Autodesk Inventor part; units mm, degrees
(part 2 of 2)
sketch "スケッチ10" plane through (0, 0, 0) normal (0, 0, 1) x (1, 0, 0)
  arc A0 (-142.506418, -9.086216) -> (-131.660668, -10.24148) centre (-136.463592, -3.843674) ccw
  line L0 (-142.506418, -9.086216) -> (-153.239213, 3.284961)
  arc A1 (-152.436991, 13.246431) -> (-153.239213, 3.284961) centre (-147.951739, 7.872185) ccw
  line L1 (-152.436991, 13.246431) -> (-136.850058, 26.255011)
  arc A2 (-136.058454, 26.82081) -> (-136.850058, 26.255011) centre (-132.685182, 21.264639) ccw
  line L2 (-136.058454, 26.82081) -> (-64.095126, 70.511318)
  arc A3 (-60.233181, 71.528052) -> (-64.095126, 70.511318) centre (-60.449397, 64.50638) ccw
  line L3 (-60.233181, 71.528052) -> (-56.416161, 71.410515)
  line L4 (-56.416161, 71.410515) -> (-62.310529, 66.98553)
  arc A4 (-62.310529, 66.98553) -> (-58.588264, 62.02723) centre (-60.449397, 64.50638) ccw
  line L5 (-58.588264, 62.02723) -> (-46.496021, 71.105048)
  line L6 (-46.496021, 71.105048) -> (-44.232954, 71.035362)
  arc A5 (-41.268818, 70.277554) -> (-44.232954, 71.035362) centre (-44.44917, 64.013691) ccw
  line L7 (-41.268818, 70.277554) -> (-66.303447, 51.483704)
  arc A6 (-66.303447, 51.483704) -> (-62.581181, 46.525404) centre (-64.442314, 49.004554) ccw
  line L8 (-62.581181, 46.525404) -> (-37.546552, 65.319255)
  arc A7 (-40.231602, 58.395617) -> (-37.546552, 65.319255) centre (-44.44917, 64.013691) ccw
  line L9 (-40.231602, 58.395617) -> (-131.660668, -10.24148)
  circle A8 centre (-147.951739, 7.872185) radius 3
  circle A9 centre (-136.463592, -3.843674) radius 3
  circle A10 centre (-84.115857, 33.578871) radius 3
  circle A11 centre (-112.106259, 12.566079) radius 3
  circle A12 centre (-77.811872, 54.579424) radius 3
  circle A13 centre (-132.685182, 21.264639) radius 3
  circle A14 centre (-105.248527, 37.922031) radius 3
  arc A15 (-133.54471, 2.112846) -> (-133.114093, 1.134364) centre (-132.555844, 1.964037) ccw
  arc A16 (-130.83606, -1.762597) -> (-133.114093, 1.134364) centre (-136.463592, -3.843674) ccw
  arc A17 (-130.83606, -1.762597) -> (-129.297772, -2.215477) centre (-129.898137, -1.415751) ccw
  line L10 (-129.297772, -2.215477) -> (-116.789492, 7.174667)
  arc A18 (-116.789492, 7.174667) -> (-116.635058, 8.630348) centre (-117.389857, 7.974392) ccw
  arc A19 (-117.147544, 9.312551) -> (-116.635058, 8.630348) centre (-112.106259, 12.566079) ccw
  arc A20 (-117.147544, 9.312551) -> (-118.117598, 9.761832) centre (-117.987758, 8.770297) ccw
  line L11 (-118.117598, 9.761832) -> (-131.933702, 7.95264)
  arc A21 (-131.933702, 7.95264) -> (-132.792729, 7.109914) centre (-131.803863, 6.961105) ccw
  line L12 (-132.792729, 7.109914) -> (-133.54471, 2.112846)
  arc A22 (-88.79909, 28.187458) -> (-88.644656, 29.643139) centre (-89.399456, 28.987184) ccw
  arc A23 (-89.943579, 32.151404) -> (-88.644656, 29.643139) centre (-84.115857, 33.578871) ccw
  arc A24 (-89.943579, 32.151404) -> (-90.713554, 32.89302) centre (-90.914866, 31.913493) ccw
  line L13 (-90.713554, 32.89302) -> (-99.456074, 34.689773)
  arc A25 (-99.456074, 34.689773) -> (-100.45612, 34.311929) centre (-99.657386, 33.710245) ccw
  arc A26 (-104.181599, 32.017655) -> (-100.45612, 34.311929) centre (-105.248527, 37.922031) ccw
  arc A27 (-104.181599, 32.017655) -> (-104.969096, 31.29467) centre (-104.003778, 31.033592) ccw
  line L14 (-104.969096, 31.29467) -> (-108.524419, 18.149127)
  arc A28 (-108.524419, 18.149127) -> (-108.208695, 17.127767) centre (-107.559102, 17.888049) ccw
  arc A29 (-107.062861, 15.816331) -> (-108.208695, 17.127767) centre (-112.106259, 12.566079) ccw
  arc A30 (-107.062861, 15.816331) -> (-105.621929, 15.558314) centre (-106.222295, 16.35804) ccw
  line L15 (-105.621929, 15.558314) -> (-88.79909, 28.187458)
  line L16 (-130.745103, 12.142434) -> (-123.324226, 13.114183)
  arc A31 (-123.324226, 13.114183) -> (-123.064726, 15.026812) centre (-123.454066, 14.105718) ccw
  line L17 (-123.064726, 15.026812) -> (-127.63835, 16.96005)
  arc A32 (-127.63835, 16.96005) -> (-128.693046, 16.785482) centre (-128.02769, 16.038956) ccw
  arc A33 (-130.949084, 15.521298) -> (-128.693046, 16.785482) centre (-132.685182, 21.264639) ccw
  arc A34 (-130.949084, 15.521298) -> (-131.6486, 14.712884) centre (-130.659734, 14.564075) ccw
  line L18 (-131.6486, 14.712884) -> (-131.863809, 13.282778)
  arc A35 (-131.863809, 13.282778) -> (-130.745103, 12.142434) centre (-130.874943, 13.133969) ccw
  arc A36 (-126.690727, 21.522538) -> (-127.791923, 24.736817) centre (-132.685182, 21.264639) ccw
  arc A37 (-126.690727, 21.522538) -> (-126.080991, 20.644427) centre (-125.691651, 21.565521) ccw
  line L19 (-126.080991, 20.644427) -> (-117.15309, 16.870668)
  arc A38 (-117.15309, 16.870668) -> (-116.098395, 17.045236) centre (-116.763751, 17.791763) ccw
  arc A39 (-113.173186, 18.470456) -> (-116.098395, 17.045236) centre (-112.106259, 12.566079) ccw
  arc A40 (-113.173186, 18.470456) -> (-112.38569, 19.19344) centre (-113.351007, 19.454519) ccw
  line L20 (-112.38569, 19.19344) -> (-108.830366, 32.338983)
  arc A41 (-108.830366, 32.338983) -> (-109.14609, 33.360343) centre (-109.795684, 32.600062) ccw
  arc A42 (-110.586613, 35.182536) -> (-109.14609, 33.360343) centre (-105.248527, 37.922031) ccw
  arc A43 (-110.586613, 35.182536) -> (-111.995259, 35.580749) centre (-111.476294, 34.725953) ccw
  line L21 (-111.995259, 35.580749) -> (-127.495344, 26.170308)
  arc A44 (-127.495344, 26.170308) -> (-127.791923, 24.736817) centre (-126.976379, 25.315513) ccw
  arc A45 (-71.858452, 55.325612) -> (-70.160292, 54.741689) centre (-70.866216, 55.449977) ccw
  arc A46 (-69.305274, 55.482332) -> (-70.160292, 54.741689) centre (-64.442314, 49.004554) ccw
  line L22 (-69.305274, 55.482332) -> (-66.550527, 57.55036)
  arc A47 (-66.550527, 57.55036) -> (-66.414464, 59.026602) centre (-67.150892, 58.350086) ccw
  arc A48 (-67.802662, 61.109398) -> (-66.414464, 59.026602) centre (-60.449397, 64.50638) ccw
  arc A49 (-67.802662, 61.109398) -> (-69.229438, 61.544813) centre (-68.710473, 60.690017) ccw
  line L23 (-69.229438, 61.544813) -> (-72.622035, 59.485093)
  arc A50 (-72.622035, 59.485093) -> (-72.918613, 58.051601) centre (-72.10307, 58.630298) ccw
  arc A51 (-71.858452, 55.325612) -> (-72.918613, 58.051601) centre (-77.811872, 54.579424) ccw
  arc A52 (-100.058689, 42.827701) -> (-100.355268, 41.394209) centre (-99.539724, 41.972905) ccw
  arc A53 (-99.420805, 39.349498) -> (-100.355268, 41.394209) centre (-105.248527, 37.922031) ccw
  arc A54 (-99.420805, 39.349498) -> (-98.650829, 38.607882) centre (-98.449518, 39.587409) ccw
  line L24 (-98.650829, 38.607882) -> (-89.908309, 36.81113)
  arc A55 (-89.908309, 36.81113) -> (-88.908264, 37.188973) centre (-89.706998, 37.790657) ccw
  arc A56 (-85.020123, 39.510338) -> (-88.908264, 37.188973) centre (-84.115857, 33.578871) ccw
  arc A57 (-85.020123, 39.510338) -> (-84.213055, 40.211408) centre (-85.170834, 40.498916) ccw
  line L25 (-84.213055, 40.211408) -> (-81.545787, 49.096917)
  arc A58 (-81.545787, 49.096917) -> (-81.833323, 50.126568) centre (-82.503565, 49.384425) ccw
  arc A59 (-83.149958, 51.839928) -> (-81.833323, 50.126568) centre (-77.811872, 54.579424) ccw
  arc A60 (-83.149958, 51.839928) -> (-84.558604, 52.238141) centre (-84.039639, 51.383346) ccw
  line L26 (-84.558604, 52.238141) -> (-100.058689, 42.827701)
  arc A61 (-137.554519, 17.758994) -> (-139.006826, 17.942469) centre (-138.366076, 17.174719) ccw
  line L27 (-139.006826, 17.942469) -> (-143.139417, 14.493481)
  arc A62 (-143.139417, 14.493481) -> (-143.180301, 12.994038) centre (-142.498667, 13.725731) ccw
  arc A63 (-141.858325, 11.317516) -> (-143.180301, 12.994038) centre (-147.951739, 7.872185) ccw
  arc A64 (-141.858325, 11.317516) -> (-140.857998, 10.818171) centre (-140.987838, 11.809706) ccw
  line L28 (-140.857998, 10.818171) -> (-136.934628, 11.331928)
  arc A65 (-136.934628, 11.331928) -> (-136.075602, 12.174654) centre (-137.064468, 12.323463) ccw
  line L29 (-136.075602, 12.174654) -> (-135.604064, 15.308119)
  arc A66 (-135.604064, 15.308119) -> (-136.03468, 16.286601) centre (-136.59293, 15.456928) ccw
  arc A67 (-137.554519, 17.758994) -> (-136.03468, 16.286601) centre (-132.685182, 21.264639) ccw
  arc A68 (-138.19969, 1.899667) -> (-137.500173, 2.708082) centre (-138.489039, 2.856891) ccw
  line L30 (-137.500173, 2.708082) -> (-137.004522, 6.001791)
  arc A69 (-137.004522, 6.001791) -> (-138.123227, 7.142135) centre (-137.993388, 6.1506) ccw
  line L31 (-138.123227, 7.142135) -> (-140.33864, 6.852031)
  arc A70 (-140.33864, 6.852031) -> (-141.176668, 6.111957) centre (-140.2088, 5.860496) ccw
  arc A71 (-144.061428, 2.05278) -> (-141.176668, 6.111957) centre (-147.951739, 7.872185) ccw
  arc A72 (-144.061428, 2.05278) -> (-144.261023, 0.566118) centre (-143.505669, 1.221436) ccw
  line L32 (-144.261023, 0.566118) -> (-143.125657, -0.742563)
  arc A73 (-143.125657, -0.742563) -> (-141.526488, -0.623878) centre (-142.370304, -0.087245) ccw
  arc A74 (-138.19969, 1.899667) -> (-141.526488, -0.623878) centre (-136.463592, -3.843674) ccw
  arc A75 (-76.907606, 48.647957) -> (-74.152214, 49.824752) centre (-77.811872, 54.579424) ccw
  arc A76 (-76.907606, 48.647957) -> (-77.714673, 47.946886) centre (-76.756895, 47.659379) ccw
  line L33 (-77.714673, 47.946886) -> (-80.381942, 39.061377)
  arc A77 (-80.381942, 39.061377) -> (-80.094406, 38.031727) centre (-79.424164, 38.77387) ccw
  arc A78 (-79.072459, 36.829123) -> (-80.094406, 38.031727) centre (-84.115857, 33.578871) ccw
  arc A79 (-79.072459, 36.829123) -> (-77.631528, 36.571106) centre (-78.231893, 37.370832) ccw
  line L34 (-77.631528, 36.571106) -> (-70.457765, 41.956551)
  arc A80 (-70.457765, 41.956551) -> (-70.331118, 43.4429) centre (-71.058131, 42.756277) ccw
  arc A81 (-72.542276, 49.029257) -> (-70.331118, 43.4429) centre (-64.442314, 49.004554) ccw
  arc A82 (-72.542276, 49.029257) -> (-74.152214, 49.824752) centre (-73.542271, 49.032306) ccw
  arc A83 (-117.147544, 9.312551) -> (-116.635058, 8.630348) centre (-112.106259, 12.566079) ccw
  arc A84 (-116.789492, 7.174667) -> (-116.635058, 8.630348) centre (-117.389857, 7.974392) ccw
  line L35 (-116.789492, 7.174667) -> (-129.297772, -2.215477)
  arc A85 (-130.83606, -1.762597) -> (-129.297772, -2.215477) centre (-129.898137, -1.415751) ccw
  arc A86 (-130.83606, -1.762597) -> (-133.114093, 1.134364) centre (-136.463592, -3.843674) ccw
  arc A87 (-133.54471, 2.112846) -> (-133.114093, 1.134364) centre (-132.555844, 1.964037) ccw
  line L36 (-133.54471, 2.112846) -> (-132.792729, 7.109914)
  arc A88 (-131.933702, 7.95264) -> (-132.792729, 7.109914) centre (-131.803863, 6.961105) ccw
  line L37 (-131.933702, 7.95264) -> (-118.117598, 9.761832)
  arc A89 (-117.147544, 9.312551) -> (-118.117598, 9.761832) centre (-117.987758, 8.770297) ccw
  arc A90 (-142.910454, 11.125713) -> (-145.546046, 13.368787) centre (-147.951739, 7.872185) ccw
  arc A91 (-145.664062, 15.139683) -> (-145.546046, 13.368787) centre (-145.145097, 14.284888) ccw
  line L38 (-145.664062, 15.139683) -> (-139.431914, 18.923356)
  arc A92 (-138.023268, 18.525143) -> (-139.431914, 18.923356) centre (-138.912949, 18.068561) ccw
  arc A93 (-138.023268, 18.525143) -> (-136.03468, 16.286601) centre (-132.685182, 21.264639) ccw
  arc A94 (-135.604064, 15.308119) -> (-136.03468, 16.286601) centre (-136.59293, 15.456928) ccw
  line L39 (-135.604064, 15.308119) -> (-136.075602, 12.174654)
  arc A95 (-136.934628, 11.331928) -> (-136.075602, 12.174654) centre (-137.064468, 12.323463) ccw
  line L40 (-136.934628, 11.331928) -> (-141.9404, 10.676432)
  arc A96 (-142.910454, 11.125713) -> (-141.9404, 10.676432) centre (-142.07024, 11.667967) ccw
  arc A97 (-110.586613, 35.182536) -> (-109.14609, 33.360343) centre (-105.248527, 37.922031) ccw
  arc A98 (-108.830366, 32.338983) -> (-109.14609, 33.360343) centre (-109.795684, 32.600062) ccw
  line L41 (-108.830366, 32.338983) -> (-112.38569, 19.19344)
  arc A99 (-113.173186, 18.470456) -> (-112.38569, 19.19344) centre (-113.351007, 19.454519) ccw
  arc A100 (-113.173186, 18.470456) -> (-116.098395, 17.045236) centre (-112.106259, 12.566079) ccw
  arc A101 (-117.15309, 16.870668) -> (-116.098395, 17.045236) centre (-116.763751, 17.791763) ccw
  line L42 (-117.15309, 16.870668) -> (-126.080991, 20.644427)
  arc A102 (-126.690727, 21.522538) -> (-126.080991, 20.644427) centre (-125.691651, 21.565521) ccw
  arc A103 (-126.690727, 21.522538) -> (-127.791923, 24.736817) centre (-132.685182, 21.264639) ccw
  arc A104 (-127.495344, 26.170308) -> (-127.791923, 24.736817) centre (-126.976379, 25.315513) ccw
  line L43 (-127.495344, 26.170308) -> (-111.995259, 35.580749)
  arc A105 (-110.586613, 35.182536) -> (-111.995259, 35.580749) centre (-111.476294, 34.725953) ccw
  arc A106 (-71.858452, 55.325612) -> (-70.160292, 54.741689) centre (-70.866216, 55.449977) ccw
  arc A107 (-71.858452, 55.325612) -> (-72.918613, 58.051601) centre (-77.811872, 54.579424) ccw
  arc A108 (-72.622035, 59.485093) -> (-72.918613, 58.051601) centre (-72.10307, 58.630298) ccw
  line L44 (-72.622035, 59.485093) -> (-69.229438, 61.544813)
  arc A109 (-67.802662, 61.109398) -> (-69.229438, 61.544813) centre (-68.710473, 60.690017) ccw
  arc A110 (-67.802662, 61.109398) -> (-66.414464, 59.026602) centre (-60.449397, 64.50638) ccw
  arc A111 (-66.550527, 57.55036) -> (-66.414464, 59.026602) centre (-67.150892, 58.350086) ccw
  line L45 (-66.550527, 57.55036) -> (-69.305274, 55.482332)
  arc A112 (-69.305274, 55.482332) -> (-70.160292, 54.741689) centre (-64.442314, 49.004554) ccw
  arc A113 (-72.542276, 49.029257) -> (-70.331118, 43.4429) centre (-64.442314, 49.004554) ccw
  arc A114 (-70.457765, 41.956551) -> (-70.331118, 43.4429) centre (-71.058131, 42.756277) ccw
  line L46 (-70.457765, 41.956551) -> (-77.631528, 36.571106)
  arc A115 (-79.072459, 36.829123) -> (-77.631528, 36.571106) centre (-78.231893, 37.370832) ccw
  arc A116 (-79.072459, 36.829123) -> (-80.094406, 38.031727) centre (-84.115857, 33.578871) ccw
  arc A117 (-80.381942, 39.061377) -> (-80.094406, 38.031727) centre (-79.424164, 38.77387) ccw
  line L47 (-80.381942, 39.061377) -> (-77.714673, 47.946886)
  arc A118 (-76.907606, 48.647957) -> (-77.714673, 47.946886) centre (-76.756895, 47.659379) ccw
  arc A119 (-76.907606, 48.647957) -> (-74.152214, 49.824752) centre (-77.811872, 54.579424) ccw
  arc A120 (-72.542276, 49.029257) -> (-74.152214, 49.824752) centre (-73.542271, 49.032306) ccw
  line L48 (-123.324226, 13.114183) -> (-130.745103, 12.142434)
  arc A121 (-131.863809, 13.282778) -> (-130.745103, 12.142434) centre (-130.874943, 13.133969) ccw
  line L49 (-131.863809, 13.282778) -> (-131.6486, 14.712884)
  arc A122 (-130.949084, 15.521298) -> (-131.6486, 14.712884) centre (-130.659734, 14.564075) ccw
  arc A123 (-130.949084, 15.521298) -> (-128.693046, 16.785482) centre (-132.685182, 21.264639) ccw
  arc A124 (-127.63835, 16.96005) -> (-128.693046, 16.785482) centre (-128.02769, 16.038956) ccw
  line L50 (-127.63835, 16.96005) -> (-123.064726, 15.026812)
  arc A125 (-123.324226, 13.114183) -> (-123.064726, 15.026812) centre (-123.454066, 14.105718) ccw
  line L51 (-99.456074, 34.689773) -> (-90.713554, 32.89302)
  arc A126 (-89.943579, 32.151404) -> (-90.713554, 32.89302) centre (-90.914866, 31.913493) ccw
  arc A127 (-89.943579, 32.151404) -> (-88.644656, 29.643139) centre (-84.115857, 33.578871) ccw
  arc A128 (-88.79909, 28.187458) -> (-88.644656, 29.643139) centre (-89.399456, 28.987184) ccw
  line L52 (-88.79909, 28.187458) -> (-105.621929, 15.558314)
  arc A129 (-107.062861, 15.816331) -> (-105.621929, 15.558314) centre (-106.222295, 16.35804) ccw
  arc A130 (-107.062861, 15.816331) -> (-108.208695, 17.127767) centre (-112.106259, 12.566079) ccw
  arc A131 (-108.524419, 18.149127) -> (-108.208695, 17.127767) centre (-107.559102, 17.888049) ccw
  line L53 (-108.524419, 18.149127) -> (-104.969096, 31.29467)
  arc A132 (-104.181599, 32.017655) -> (-104.969096, 31.29467) centre (-104.003778, 31.033592) ccw
  arc A133 (-104.181599, 32.017655) -> (-100.45612, 34.311929) centre (-105.248527, 37.922031) ccw
  arc A134 (-99.456074, 34.689773) -> (-100.45612, 34.311929) centre (-99.657386, 33.710245) ccw
  line L54 (-100.058689, 42.827701) -> (-84.558604, 52.238141)
  arc A135 (-83.149958, 51.839928) -> (-84.558604, 52.238141) centre (-84.039639, 51.383346) ccw
  arc A136 (-83.149958, 51.839928) -> (-81.833323, 50.126568) centre (-77.811872, 54.579424) ccw
  arc A137 (-81.545787, 49.096917) -> (-81.833323, 50.126568) centre (-82.503565, 49.384425) ccw
  line L55 (-81.545787, 49.096917) -> (-84.213055, 40.211408)
  arc A138 (-85.020123, 39.510338) -> (-84.213055, 40.211408) centre (-85.170834, 40.498916) ccw
  arc A139 (-85.020123, 39.510338) -> (-88.908264, 37.188973) centre (-84.115857, 33.578871) ccw
  arc A140 (-89.908309, 36.81113) -> (-88.908264, 37.188973) centre (-89.706998, 37.790657) ccw
  line L56 (-89.908309, 36.81113) -> (-98.650829, 38.607882)
  arc A141 (-99.420805, 39.349498) -> (-98.650829, 38.607882) centre (-98.449518, 39.587409) ccw
  arc A142 (-99.420805, 39.349498) -> (-100.355268, 41.394209) centre (-105.248527, 37.922031) ccw
  arc A143 (-100.058689, 42.827701) -> (-100.355268, 41.394209) centre (-99.539724, 41.972905) ccw
  line L57 (-141.421042, 6.710292) -> (-138.123227, 7.142135)
  arc A144 (-137.004522, 6.001791) -> (-138.123227, 7.142135) centre (-137.993388, 6.1506) ccw
  line L58 (-137.004522, 6.001791) -> (-137.500173, 2.708082)
  arc A145 (-138.19969, 1.899667) -> (-137.500173, 2.708082) centre (-138.489039, 2.856891) ccw
  arc A146 (-138.19969, 1.899667) -> (-142.031716, -1.608501) centre (-136.463592, -3.843674) ccw
  arc A147 (-143.581885, -2.018871) -> (-142.031716, -1.608501) centre (-142.959736, -1.235972) ccw
  line L59 (-143.581885, -2.018871) -> (-146.594315, 0.375026)
  arc A148 (-146.254963, 2.117105) -> (-146.594315, 0.375026) centre (-145.972167, 1.157925) ccw
  arc A149 (-146.254963, 2.117105) -> (-142.242708, 6.02639) centre (-147.951739, 7.872185) ccw
  arc A150 (-141.421042, 6.710292) -> (-142.242708, 6.02639) centre (-141.291203, 5.718757) ccw
  circle A151 centre (-132.685182, 21.264639) radius 3
  circle A152 centre (-105.248527, 37.922031) radius 3
  circle A153 centre (-84.115857, 33.578871) radius 3
  circle A154 centre (-77.811872, 54.579424) radius 3
  circle A155 centre (-112.106259, 12.566079) radius 3
  circle A156 centre (-136.463592, -3.843674) radius 3
  circle A157 centre (-147.951739, 7.872185) radius 3
  line L60 (-62.310529, 66.98553) -> (-56.416161, 71.410515)
  line L61 (-56.416161, 71.410515) -> (-60.233181, 71.528052)
  arc A158 (-60.233181, 71.528052) -> (-64.095126, 70.511318) centre (-60.449397, 64.50638) ccw
  line L62 (-64.095126, 70.511318) -> (-153.154364, 16.44151)
  arc A159 (-153.154364, 16.44151) -> (-154.18878, 0.023621) centre (-147.951739, 7.872185) ccw
  line L63 (-154.18878, 0.023621) -> (-141.440781, -10.106867)
  arc A160 (-141.440781, -10.106867) -> (-131.660668, -10.24148) centre (-136.463592, -3.843674) ccw
  line L64 (-131.660668, -10.24148) -> (-40.231602, 58.395617)
  arc A161 (-40.231602, 58.395617) -> (-37.546552, 65.319255) centre (-44.44917, 64.013691) ccw
  line L65 (-37.546552, 65.319255) -> (-62.581181, 46.525404)
  arc A162 (-66.303447, 51.483704) -> (-62.581181, 46.525404) centre (-64.442314, 49.004554) ccw
  line L66 (-66.303447, 51.483704) -> (-41.268818, 70.277554)
  arc A163 (-41.268818, 70.277554) -> (-44.232954, 71.035362) centre (-44.44917, 64.013691) ccw
  line L67 (-44.232954, 71.035362) -> (-46.496021, 71.105048)
  line L68 (-46.496021, 71.105048) -> (-58.588264, 62.02723)
  arc A164 (-62.310529, 66.98553) -> (-58.588264, 62.02723) centre (-60.449397, 64.50638) ccw
  point P0 (0, 0)
  point P1 (0, 0)
  point P2 (-136.058454, 26.82081)
  point P3 (-140.857998, 10.818171)
  point P4 (-137.554519, 17.758994)
  point P5 (-141.526488, -0.623878)
  constraints: 152 point on circle, 83 centre point, 70 end point, 314 other
extrude "押し出し8" cut sketch "スケッチ10" against normal blind 10 contours A0 L63 A159 L62 A2 L1 A1 L0
extrude "押し出し9" add sketch "スケッチ10" against normal blind 5 contours A61 L27 A62 A63 A64 L40 A96 A90 A91 L38 A92 A93 | A146 A147 L59 A148 A149 A150 L57 A70 A71 A72 L32 A73
equation "\"d30\" = 0.5 * d29"
equation "\"d57\" = d59"
equation "\"d58\" = d59"
equation "\"d61\" = d60"
equation "\"d62\" = d60"
equation "\"d63\" = d62"
